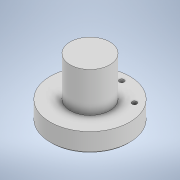
# Autodesk Inventor part: Część4
Saved by Autodesk Inventor 2021 (Build 250183000, 183)
## iProperties
Created: 2023-09-22
Part Number: Część4
Material: Ogólny
Document SubType Name: Modeling
Designer: Jakub
Density: 1 g/cm^3
Appearance: Domyślna
Author: Jakub
Autodesk Inventor part; units mm, degrees
ref_plane "YZ Plane" through (0, 0, 0) normal (1, 0, 0) x (0, 1, 0)
ref_plane "XZ Plane" through (0, 0, 0) normal (0, 1, 0) x (-1, 0, 0)
ref_plane "XY Plane" through (0, 0, 0) normal (0, 0, 1) x (1, 0, 0)
sketch "Szkic1" plane through (0, 0, 0) normal (0, 1, 0) x (-1, 0, 0)
  circle A0 centre (0, 0) radius 25
  dimension "d0" = 50
  constraints: 1 centre point, 1 coincident
  measures "d0" diameter of A0
extrude "Wyciągnięcie proste1" add sketch "Szkic1" along normal blind 12
sketch "Szkic2" plane through (0, 0, 0) normal (0, -1, 0) x (1, 0, 0)
  circle A0 centre (0, 0) radius 6
  dimension "d3" = 12
  constraints: 1 centre point, 1 coincident
  measures "d3" diameter of A0
extrude "Wyciągnięcie proste2" add sketch "Szkic2" along normal blind 3
sketch "Szkic3" plane through (0, 12, 0) normal (0, 1, 0) x (1, 0, 0)
  circle A0 centre (0, 0) radius 12.5
  dimension "d6" = 25
  constraints: 1 centre point, 1 coincident
  measures "d6" diameter of A0
extrude "Wyciągnięcie proste3" add sketch "Szkic3" along normal blind 25
chamfer "Faza1" distance 1 angle 45 1 edges at (-6, -3, 0)
chamfer "Faza2" distance 1 angle 45 1 edges at (25, 0, 0)
sketch "Szkic6" plane through (0, 0, 0) normal (0, -1, 0) x (1, 0, 0)
  circle A0 centre (0, 0) radius 20
  circle A1 centre (-16, -12) radius 1.5
  dimension "d16" = 40
  dimension "d17" = 3
  constraints: 2 centre point, 1 coincident
  measures "d16" diameter of A0
  measures "d17" diameter of A1
extrude "Wyciągnięcie proste4" cut sketch "Szkic6" against normal blind 25 contours A1 A0 | A0 A1 picked at (-15.6226, -11.6657) picked at (-16.3566, -12.3446)
sketch "Szkic7" plane through (0, 0, 0) normal (0, -1, 0) x (1, 0, 0)
  circle A0 centre (0, 0) radius 5 projected
  circle A1 centre (0, 0) radius 20
  circle A2 centre (16, -12) radius 1.5
  dimension "d20" = 40
  dimension "d21" = 3
  constraints: 1 centre point, 1 coincident, 3 other
  measures "d21" diameter of A2
extrude "Wyciągnięcie proste5" cut sketch "Szkic7" against normal blind 25 contours A2 A1 | A1 A2 picked at (15.5641, -11.7467) picked at (16.3868, -12.3102)
sketch "Szkic9" plane through (0, 0, 0) normal (0, -1, 0) x (1, 0, 0)
  circle A0 centre (0, -20) radius 1.5
  point P0 (0, 0)
  dimension "d25" = 3
  constraints: 1 centre point
  measures "d25" diameter of A0
extrude "Wyciągnięcie proste6" cut sketch "Szkic9" against normal blind 25
